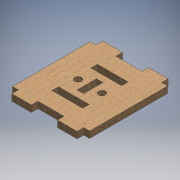
# Autodesk Inventor part: LightDiskSupport
Saved by Autodesk Inventor 2016 (Build 200138000, 138)
## iProperties
Created: 2015-12-14
Part Number: LightDiskSupport
Material: MDF Medium Density Fiberboard
Document SubType Name: Modeling
Designer: momem
Density: 0.8 g/cm^3
Appearance: Cardboard - Corrugated
Author: momem
Autodesk Inventor part; units mm, degrees
ref_plane "YZ Plane" through (0, 0, 0) normal (1, 0, 0) x (0, 1, 0)
ref_plane "XZ Plane" through (0, 0, 0) normal (0, 1, 0) x (-1, 0, 0)
ref_plane "XY Plane" through (0, 0, 0) normal (0, 0, 1) x (1, 0, 0)
sketch "Sketch1" plane through (0, 0, 0) normal (0, 0, 1) x (1, 0, 0)
  line L0 (-37.5, 37.9177) -> (-31.7388, 37.9177)
  line L1 (37.5, 37.9177) -> (37.5, -37.9177)
  line L2 (37.5, -37.9177) -> (31.7388, -37.9177)
  line L3 (-37.5, -37.9177) -> (-37.5, 37.9177)
  line L4 (-31.7388, 37.9177) -> (-31.7388, 44.3077)
  line L5 (-31.7388, 44.3077) -> (-12.78, 44.3077)
  line L6 (-12.78, 44.3077) -> (-12.78, 37.9177)
  line L7 (0, 37.9177) -> (0, -37.9177) construction
  line L8 (-37.5, 0) -> (37.5, 0) construction
  line L9 (-12.78, 37.9177) -> (12.78, 37.9177)
  line L10 (31.7388, 37.9177) -> (31.7388, 44.3077)
  line L11 (31.7388, 44.3077) -> (12.78, 44.3077)
  line L12 (12.78, 44.3077) -> (12.78, 37.9177)
  line L13 (-31.7388, -37.9177) -> (-31.7388, -44.3077)
  line L14 (-31.7388, -44.3077) -> (-12.78, -44.3077)
  line L15 (-12.78, -44.3077) -> (-12.78, -37.9177)
  line L16 (12.78, -44.3077) -> (12.78, -37.9177)
  line L17 (31.7388, -44.3077) -> (12.78, -44.3077)
  line L18 (31.7388, -37.9177) -> (31.7388, -44.3077)
  line L19 (31.7388, 37.9177) -> (37.5, 37.9177)
  line L20 (-31.7388, -37.9177) -> (-37.5, -37.9177)
  line L21 (12.78, -37.9177) -> (-12.78, -37.9177)
  line L22 (-14.945, 15.7638) -> (14.945, 15.7638)
  line L23 (14.945, 15.7638) -> (14.945, 22.1538)
  line L24 (14.945, 22.1538) -> (-14.945, 22.1538)
  line L25 (-14.945, 22.1538) -> (-14.945, 15.7638)
  line L26 (-14.945, -15.7638) -> (14.945, -15.7638)
  line L27 (14.945, -15.7638) -> (14.945, -22.1538)
  line L28 (14.945, -22.1538) -> (-14.945, -22.1538)
  line L29 (-14.945, -22.1538) -> (-14.945, -15.7638)
  line L30 (-3.195, 9.4794) -> (3.195, 9.4794)
  line L31 (3.195, 9.4794) -> (3.195, -9.4794)
  line L32 (3.195, -9.4794) -> (-3.195, -9.4794)
  line L33 (-3.195, -9.4794) -> (-3.195, 9.4794)
  line L34 (-14.945, 18.9588) -> (14.945, 18.9588) construction
  circle A0 centre (-11.6112, 0) radius 3.3338
  circle A1 centre (11.6112, 0) radius 3.3338
  point P0 (0, 0)
  point P1 (0, 22.1538)
  point P2 (3.195, 0)
  point P3 (0, 0)
  point P4 (0, 9.4794)
  point P5 (0, 0)
  point P6 (-22.2594, -44.3077)
  dimension "d0" = 75
  dimension "d1" = 75.8353
  dimension "d2" = 18.9588
  dimension "d3" = 6.39
  dimension "d4" = 12.78
  dimension "d21" = 6.39
  dimension "d22" = 29.89
  dimension "d24" = 18.9588
  dimension "d25" = 6.39
  dimension "d30" = 37.9177
  dimension "d41" = 6.6675
  constraints: 70 end point, 17 symmetric about line, 14 parallel, 12 perpendicular, 11 midpoint, 5 horizontal, 3 vertical alignment, 2 centre point, 2 horizontal alignment, 2 point on line, 1 coincident, 1 collinear, 1 tangent, 1 other
  measures "d0" distance of L0.start L1.start
  measures "d1" distance of L1.start L1.end
  measures "d2" distance of L4.end L5.end
  measures "d3" distance of L5.end L6.end
  measures "d4" distance between parallel lines of L6 L7
  measures "d21" distance of L24.end L22.start
  measures "d22" distance of L23.end L24.end
  measures "d24" distance of L30.end L31.end
  measures "d25" distance of L31.end L32.end
  measures "d30" distance between parallel lines of L28 L22
  measures "d41" diameter of A0
extrude "Extrusion4" add sketch "Sketch1" along normal blind 6.39
equation "\"d1\" = DiskGap"
equation "\"d2\" = 0.25 * DiskGap"
equation "\"d3\" = WoodThickness"
equation "\"d4\" = 2 * WoodThickness"
equation "\"d21\" = WoodThickness"
equation "\"d22\" = 0.5 * ColumnWidth"
equation "\"d24\" = 0.25 * DiskGap"
equation "\"d25\" = WoodThickness"
equation "\"d30\" = 0.5 * DiskGap"
equation "\"d42\" = WoodThickness"
equation "\"DiskGap\" = 75.835317"
equation "\"WoodThickness\" = 6.39"
equation "\"ColumnWidth\" = 59.78"
body "Solid4"
